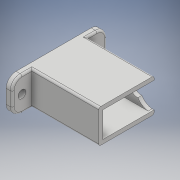
# Autodesk Inventor part: Support bas servomoteur
Saved by Autodesk Inventor 2017 (Build 210142000, 142)
## iProperties
Part Number: Support bas servomoteur
Material: Générique
Document SubType Name: Modeling
Designer: Geoff
Density: 1 g/cm^3
Appearance: Par défaut
Author: Geoff
Autodesk Inventor part; units mm, degrees
ref_plane "YZ Plane" through (0, 0, 0) normal (1, 0, 0) x (0, 1, 0)
ref_plane "XZ Plane" through (0, 0, 0) normal (0, 1, 0) x (-1, 0, 0)
ref_plane "XY Plane" through (0, 0, 0) normal (0, 0, 1) x (1, 0, 0)
sketch "Esquisse5" plane through (0, 0, 0) normal (1, 0, 0) x (0, 1, 0)
  line L0 (0, 0) -> (28, 0)
  line L1 (28, 0) -> (28, -17)
  line L2 (28, -17) -> (0, -17)
  line L3 (0, -17) -> (0, 0)
  line L4 (0, 0) -> (0, -2)
  line L5 (0, -2) -> (2, -2)
  line L6 (28, -17) -> (28, -15)
  line L7 (28, -15) -> (26, -15)
  line L8 (26, -15) -> (2, -15)
  line L9 (2, -15) -> (2, -2)
  line L10 (2, -2) -> (26, -2)
  line L11 (26, -2) -> (26, -15)
  dimension "d20" = 28
  dimension "d21" = 17
  dimension "d22" = 2
  dimension "d23" = 2
  dimension "d24" = 2
  dimension "d25" = 2
  constraints: 24 end point, 4 parallel, 4 perpendicular, 2 horizontal, 2 point on line
  measures "d20" distance of L1.end L2.end
  measures "d21" distance of L0.end L1.end
  measures "d22" distance of L0.start L4.end
  measures "d23" distance of L4.end L5.end
  measures "d24" distance of L1.end L6.end
  measures "d25" distance of L6.end L7.end
extrude "Extrusion4" add sketch "Esquisse5" along normal blind 23.4 contours L0 L1 L7 L11 L10 L5 L3 | L5 L9 L8 L7 L1 L2 L3
sketch "Esquisse6" plane through (0, 0, 0) normal (-1, 0, 0) x (0, 0, 1)
  line L0 (-15, 2) -> (-2, 2) projected
  line L1 (-2, 2) -> (-2, 26) projected
  line L2 (-15, 2) -> (-2, 2)
  line L3 (-2, 2) -> (-2, 26)
  line L4 (-2, 26) -> (-15, 26)
  line L5 (-15, 26) -> (-15, 2)
  point P0 (0, 0)
  constraints: 8 end point, 2 parallel, 1 horizontal, 1 perpendicular
extrude "Extrusion5" add sketch "Esquisse6" against normal blind 2
sketch "Esquisse7" plane through (2, 0, 0) normal (1, 0, 0) x (0, 0, -1)
  line L0 (15, 2) -> (2, 2)
  line L1 (2, 2) -> (2, 19.4)
  line L2 (2, 2) -> (2, 26)
  line L3 (2, 19.4) -> (2, 21.5)
  line L4 (2, 21.5) -> (2, 26)
  line L5 (2, 21.5) -> (2, 26)
  line L6 (15, 2) -> (2, 2)
  line L7 (2, 2) -> (2, 19.4)
  line L8 (2, 19.4) -> (15, 19.4)
  line L9 (15, 19.4) -> (15, 2)
  line L10 (2, 26) -> (15, 26)
  line L11 (15, 26) -> (2, 26)
  line L12 (2, 26) -> (2, 21.5)
  line L13 (2, 21.5) -> (15, 21.5)
  line L14 (15, 21.5) -> (15, 26)
  point P0 (0, 0)
  dimension "d30" = 17.4
  dimension "d31" = 2.1
  constraints: 30 end point, 4 parallel, 2 collinear, 2 horizontal, 2 perpendicular, 2 point on line
  measures "d30" distance of L0.end L1.end
  measures "d31" distance of L1.end L3.end
extrude "Extrusion6" add sketch "Esquisse7" along normal blind 4.5
sketch "Esquisse8" plane through (6.5, 0, 0) normal (1, 0, 0) x (0, 0, -1)
  line L0 (15, 26) -> (15, 2) projected
  line L1 (2, 2) -> (15, 2)
  line L2 (15, 2) -> (15, 10)
  line L3 (15, 10) -> (2, 10)
  line L4 (2, 10) -> (2, 2)
  point P0 (0, 0)
  dimension "d34" = 8
  constraints: 8 end point, 2 parallel, 1 horizontal, 1 perpendicular, 1 point on line
  measures "d34" distance of L2.end L1.end
extrude "Extrusion7" cut sketch "Esquisse8" against normal up to next
sketch "Esquisse9" plane through (0, 28, 0) normal (0, 1, 0) x (1, 0, 0)
  line L0 (22.4357, 15) -> (23.4, 15)
  line L1 (22.4357, 2) -> (23.4, 2)
  arc A0 (23.4, 15) -> (23.4, 2) centre (22.9179, 8.5) ccw
  line L2 (23.4, 2) -> (23.4, 15)
  line L3 (23.4, 15) -> (23.4, 2)
  line L4 (23.4, 2) -> (23.4, 15) projected
  line L5 (23.4, 0) -> (23.4, 2)
  point P0 (0, 0)
  constraints: 10 end point, 4 point on circle, 1 centre point, 1 collinear, 1 perpendicular
extrude "Extrusion8" cut sketch "Esquisse9" against normal blind 4.5 contours L0 L2 L1 A0
sketch "Esquisse10" plane through (6.5, 26, -15) normal (0, -1, 0) x (1, 0, 0)
  line L0 (0, 13) -> (0, 0) projected
  line L1 (0, 6.5) -> (7, 6.5)
  line L2 (7, 6.5) -> (10.25, 6.5)
  circle A0 centre (10.25, 6.5) radius 3.25
  point P0 (-6.5, 15)
  dimension "d39" = 7
  dimension "d41" = 6.5
  constraints: 4 end point, 2 coincident, 2 horizontal, 1 centre point, 1 midpoint
  measures "d39" distance of L1.start L1.end
  measures "d41" diameter of A0
extrude "Extrusion9" cut sketch "Esquisse10" against normal up to next
sketch "Esquisse11" plane through (0, 0, 0) normal (-1, 0, 0) x (0, 0, 1)
  line L0 (-17, 28) -> (-15, 28) projected
  line L1 (0, 0) -> (-17, 0)
  line L2 (-17, 0) -> (-17, 28)
  line L3 (-17, 28) -> (0, 28)
  line L4 (0, 28) -> (0, 0)
  line L5 (-2, 2) -> (-2, 28) projected
  line L6 (-15, 26) -> (-15, 21.5) projected
  line L7 (-2, 2) -> (-15, 2)
  line L8 (-15, 2) -> (-15, 26)
  line L9 (-15, 26) -> (-2, 26)
  line L10 (-2, 26) -> (-2, 2)
  constraints: 16 end point, 4 parallel, 2 horizontal, 2 perpendicular
extrude "Extrusion10" add sketch "Esquisse11" along normal blind 13.5
sketch "Esquisse12" plane through (-13.5, 0, 0) normal (-1, 0, 0) x (0, 0, 1)
  line L0 (0, 0) -> (-17, 0)
  line L1 (-17, 0) -> (-17, -10)
  line L2 (-17, -10) -> (0, -10)
  line L3 (0, -10) -> (0, 0)
  line L4 (0, 28) -> (0, 0) projected
  line L5 (0, 28) -> (-17, 28)
  line L6 (-17, 28) -> (-17, 38)
  line L7 (-17, 38) -> (0, 38)
  line L8 (0, 38) -> (0, 28)
  dimension "d46" = 17
  dimension "d47" = 10
  dimension "d50" = 17
  dimension "d51" = 10
  constraints: 16 end point, 4 parallel, 2 horizontal, 2 perpendicular
  measures "d46" distance of L2.end L1.end
  measures "d47" distance of L1.end L0.end
  measures "d50" distance of L6.end L7.end
  measures "d51" distance of L5.end L6.end
extrude "Extrusion11" add sketch "Esquisse12" against normal blind 3
fillet "Congé1" radius 5 1 edges at (-12, 38, -17)
fillet "Congé2" radius 5 3 edges at (-12, 38, 0) (-12, -10, -17) (-12, -10, 0)
sketch "Esquisse13" plane through (-10.5, 0, 0) normal (1, 0, 0) x (0, 0, -1)
  line L0 (5, -10) -> (12, -10) projected
  line L1 (8.5, -10) -> (8.5, -5)
  line L2 (8.5, -5) -> (8.5, 33)
  circle A0 centre (8.5, -5) radius 2
  circle A1 centre (8.5, 33) radius 2
  point P0 (0, 0)
  dimension "d54" = 5
  dimension "d55" = 38
  dimension "d56" = 4
  dimension "d57" = 4
  constraints: 4 end point, 2 centre point, 2 coincident, 1 midpoint, 1 point on line, 1 vertical
  measures "d54" distance of L1.start L1.end
  measures "d55" distance of L1.end L2.end
  measures "d56" diameter of A0
  measures "d57" diameter of A1
extrude "Extrusion12" cut sketch "Esquisse13" against normal up to next
fillet "Congé3" radius 1 14 edges at (6.45, 28, -17) (6.45, 0, -17) (6.45, 0, 0) (6.45, 28, 0) (-10.5, 36.5355, -15.5355) (-10.5, 38, -8.5) (-10.5, 36.5355, -1.4645) (-10.5, 30.5, 0) (-10.5, 30.5, -17) (-10.5, -8.5355, -15.5355) (-10.5, -10, -8.5) (-10.5, -8.5355, -1.4645) (-10.5, -2.5, 0) (-10.5, -2.5, -17)
